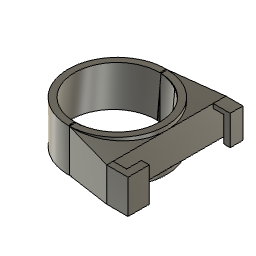
ring-updated (1) (Autodesk Fusion 360 design; units mm, degrees)
Autodesk Fusion 360 part; units mm, degrees
sketch "Sketch1" plane through (0, 0, 0) normal (0, 0, 1) x (1, 0, 0)
  circle A0 centre (0, 0) radius 10
  circle A1 centre (0, 0) radius 11.5
  dimension "d1" = 20
  dimension "d2" = 23
  constraint coincident A0.centre A1.centre
  constraint concentric A0 A1
  measures "d1" diameter of A0
  measures "d2" diameter of A1
extrude "Extrude1" add sketch "Sketch1" along normal blind 10 contours A1 picked at (10.957185, -0.571329)
ref_plane "WorkPlane1" through (11.5, 0, 5.189024) normal (1, 0, 0) x (0, -1, 0)
ref_plane "WorkPlane2" through (0, 0, 0) normal (1, 0, 0) x (0, 1, 0)
sketch "Sketch3" plane through (0, 0, 0) normal (1, 0, 0) x (0, 1, 0)
  line L0 (-11.442361, 10.021666) -> (11.442361, 10.021666)
  line L1 (11.442361, 10.021666) -> (11.442361, 0)
  line L2 (11.442361, 0) -> (-11.442361, 0)
  line L3 (-11.442361, 0) -> (-11.442361, 10.021666)
  constraint horizontal L0
  constraint vertical L1
  constraint horizontal L2
  constraint vertical L3
sketch "Sketch4" plane through (11.5, 0, 0) normal (1, 0, 0) x (0, 1, 0)
  line L0 (-14, 9) -> (14, 9)
  line L1 (14, 9) -> (14, 1)
  line L2 (14, 1) -> (-14, 1)
  line L3 (-14, 1) -> (-14, 9)
  line L4 (-14, 9) -> (14, 1) construction
  line L5 (14, 9) -> (-14, 1) construction
  point P0 (0, 5)
  dimension "d11" = 28
  dimension "d12" = 8
  constraint horizontal L0
  constraint perpendicular L0 L1
  constraint parallel L0 L2
  constraint parallel L1 L3
  constraint coincident L4 P0
  constraint coincident L5 P0
  measures "d11" distance of L1.end L2.end
  measures "d12" distance of L0.end L1.end
loft "Loft1" add profiles "Sketch3", "Sketch4" section 1 contours L0 L1 L2 L3 picked at (-3.81412, 6.68111) section 2 contours L0 L1 L2 L3 picked at (-4.666667, 6.333333)
sketch "Sketch5" plane through (0.883357, 0, 9.943188) normal (0.088492, 0, 0.996077) x (0, 1, 0)
  line L0 (-11.496599, 0.642006) -> (-9.997026, 0.642006)
  ellipse E0 centre (0, 0.886837) end of major axis (0, -9.152549) minor radius 10 (-9.997026, 0.642006) -> (9.997026, 0.642006) ccw
  line L1 (9.997026, 0.642006) -> (11.496599, 0.642006)
  line L2 (11.496599, 0.642006) -> (11.442361, 0.886837)
  line L3 (11.442361, 0.886837) -> (-11.442361, 0.886837)
  line L4 (-11.442361, 0.886837) -> (-11.496599, 0.642006)
  circle A0 centre (0, 0.886837) radius 10.008325
  constraint concentric E0 A0
extrude "Extrude3" cut sketch "Sketch5" against normal blind 15 contours E0 L3 A0 | L3 A0 picked at (-3.308097, -0.1074) picked at (0.249308, 4.213617)
sketch "Sketch7" plane through (11.5, 0, 0) normal (1, 0, 0) x (0, 1, 0)
  line L0 (0, 9) -> (-14, 9)
  line L1 (-14, 9) -> (-14, 1)
  line L2 (-14, 1) -> (0, 1)
  line L3 (0, 1) -> (14, 1)
  line L4 (14, 1) -> (14, 9)
  line L5 (14, 9) -> (0, 9)
  line L6 (11, 9) -> (14, 9)
  line L7 (14, 9) -> (14, 2)
  line L8 (14, 2) -> (11, 2)
  line L9 (11, 2) -> (11, 9)
  dimension "d15" = 7
  constraint horizontal L6
  constraint vertical L7
  constraint horizontal L8
  constraint vertical L9
  constraint coincident L5 L6.start
  measures "d15" distance of L6.start L8.end
extrude "Extrude4" add sketch "Sketch7" along normal blind 4 contours L4 L5 L6 L7 L8 L9 picked at (12, 6.666667)
sketch "Sketch8" plane through (0, 11, 0) normal (0, -1, 0) x (1, 0, 0)
  line L0 (11.5, 9) -> (11.5, 2)
  line L1 (11.5, 2) -> (15.5, 2)
  line L2 (15.5, 2) -> (15.5, 9)
  line L3 (15.5, 9) -> (11.5, 9)
  line L4 (11.5, 8.003479) -> (14, 8.003479)
  line L5 (14, 8.003479) -> (14, 2)
  line L6 (14, 2) -> (11.5, 2)
  line L7 (11.5, 2) -> (11.5, 8.003479)
  constraint horizontal L4
  constraint vertical L5
  constraint horizontal L6
  constraint vertical L7
  constraint coincident L1 L5.end
extrude "Extrude5" cut sketch "Sketch8" against normal blind 12 contours L0 L1 L4 L5 L6 L7 picked at (13.166667, 4.00116)
sketch "Sketch9" plane through (11.5, 0, 0) normal (1, 0, 0) x (0, 1, 0)
  line L0 (11, 8.003479) -> (11, 9)
  line L1 (11, 9) -> (0, 9)
  line L2 (0, 9) -> (-14, 9)
  line L3 (-14, 9) -> (-14, 1)
  line L4 (-14, 1) -> (0, 1)
  line L5 (0, 1) -> (14, 1)
  line L6 (14, 1) -> (14, 8.003479)
  line L7 (14, 8.003479) -> (11, 8.003479)
  line L8 (-14, 9) -> (-9, 9)
  line L9 (-9, 9) -> (-9, 1)
  line L10 (-9, 1) -> (-14, 1)
  line L11 (-14, 1) -> (-14, 9)
  constraint horizontal L8
  constraint vertical L9
  constraint horizontal L10
  constraint vertical L11
  constraint coincident L4 L9.end
  constraint coincident L2.end L3.start
extrude "Extrude6" add sketch "Sketch9" along normal blind 5 contours L2 L3 L4 L8 L9 L10 L11 picked at (-12.333333, 6.333333)
sketch "Sketch10" plane through (0, -9, 0) normal (0, 1, 0) x (-1, 0, 0)
  line L0 (-11.5, 1) -> (-11.5, 9)
  line L1 (-11.5, 9) -> (-16.5, 9)
  line L2 (-16.5, 9) -> (-16.5, 1)
  line L3 (-16.5, 1) -> (-11.5, 1)
  line L4 (-11.5, 1) -> (-14.676721, 1)
  line L5 (-14.676721, 1) -> (-14.676721, 9)
  line L6 (-14.676721, 9) -> (-11.5, 9)
  line L7 (-11.5, 9) -> (-11.5, 1)
  constraint horizontal L4
  constraint vertical L5
  constraint horizontal L6
  constraint vertical L7
  constraint coincident L0.start L3.end
extrude "Extrude7" cut sketch "Sketch10" against normal blind 3.5 contours L0 L1 L3 L4 L5 L6 L7 picked at (-12.558907, 3.666667)
sketch "Sketch12" plane through (0, 0, 1) normal (0, 0, -1) x (1, 0, 0)
  line L0 (11.5, 12.5) -> (14.676721, 12.5)
  line L1 (14.676721, 12.5) -> (14.676721, 9)
  line L2 (14.676721, 9) -> (16.5, 9)
  line L3 (16.5, 9) -> (16.5, 14)
  line L4 (16.5, 14) -> (11.5, 14)
  line L5 (11.5, 14) -> (11.5, 12.5)
  line L6 (11.5, 14) -> (16.5, 14)
  line L7 (16.5, 14) -> (16.5, 9)
  line L8 (16.5, 9) -> (11.5, 9)
  line L9 (11.5, 9) -> (11.5, 14)
  constraint horizontal L6
  constraint vertical L7
  constraint horizontal L8
  constraint vertical L9
  constraint coincident L2.end L3.start
  constraint coincident L4.end L5.start
extrude "Extrude8" add sketch "Sketch12" against normal blind 1 contours L0 L1 L8 L9 picked at (12.558907, 10.166667)
